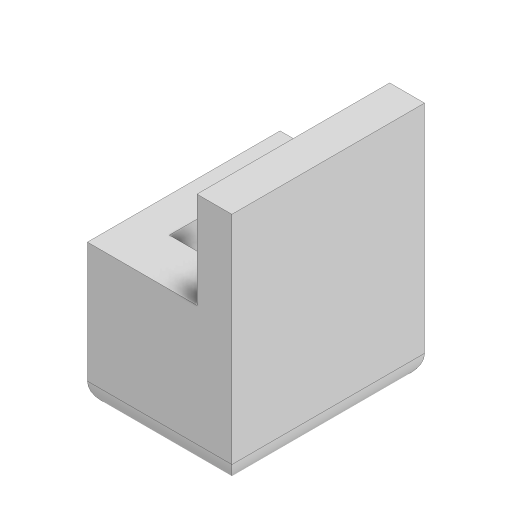
# Autodesk Inventor part: SEGURO DE GUIA DE TAPA PRINCIPAL
Saved by Autodesk Inventor 2024 (Build 280153000, 153)
## iProperties
Created: 2024-09-04
Part Number: SEGURO DE GUIA DE TAPA PRINCIPAL
Material: Generic
Document SubType Name: Modeling
Designer: Jhuliams
Density: 1 g/cm^3
Appearance: Default
Author: Jhuliams
Autodesk Inventor part; units mm, degrees
ref_plane "YZ Plane" through (0, 0, 0) normal (1, 0, 0) x (0, 1, 0)
ref_plane "XZ Plane" through (0, 0, 0) normal (0, 1, 0) x (-1, 0, 0)
ref_plane "XY Plane" through (0, 0, 0) normal (0, 0, 1) x (1, 0, 0)
sketch "Sketch1" plane through (0, 0, 0) normal (0, 1, 0) x (-1, 0, 0)
  line L0 (15, 20) -> (-15, 20)
  line L1 (-15, 20) -> (-15, -20)
  line L2 (-15, -20) -> (15, -20)
  line L3 (15, -20) -> (15, 20)
  line L4 (15, 20) -> (-15, -20) construction
  line L5 (-15, 20) -> (15, -20) construction
  point P0 (0, 0)
  dimension "d0" = 30
  dimension "d1" = 40
  constraints: 12 end point, 2 midpoint, 2 parallel, 1 horizontal, 1 perpendicular
  measures "d0" distance of L2.end L1.end
  measures "d1" distance of L1.end L0.end
extrude "Extrusion1" add sketch "Sketch1" along normal blind 50
sketch "Sketch2" plane through (0, 50, 0) normal (0, 1, 0) x (1, 0, 0)
  line L0 (-7.75, -25.4) -> (7.75, -25.4)
  line L1 (7.75, -25.4) -> (7.75, 25.4)
  line L2 (7.75, 25.4) -> (-7.75, 25.4)
  line L3 (-7.75, 25.4) -> (-7.75, -25.4)
  line L4 (-7.75, -25.4) -> (7.75, 25.4) construction
  line L5 (7.75, -25.4) -> (-7.75, 25.4) construction
  point P0 (0, 0)
  dimension "d4" = 15.5
  constraints: 12 end point, 2 midpoint, 2 parallel, 1 horizontal, 1 perpendicular
  measures "d4" distance of L2.end L1.end
extrude "Extrusion2" cut sketch "Sketch2" against normal blind 20
sketch "Sketch3" plane through (0, 30, 0) normal (0, 1, 0) x (1, 0, 0)
  line L0 (-7.75, -10.25) -> (7.75, -10.25)
  line L1 (7.75, -10.25) -> (7.75, 10.25)
  line L2 (7.75, 10.25) -> (-7.75, 10.25)
  line L3 (-7.75, 10.25) -> (-7.75, -10.25)
  line L4 (-7.75, -10.25) -> (7.75, 10.25) construction
  line L5 (7.75, -10.25) -> (-7.75, 10.25) construction
  point P0 (0, 0)
  dimension "d7" = 15.5
  dimension "d8" = 20.5
  constraints: 12 end point, 2 midpoint, 2 parallel, 1 horizontal, 1 perpendicular
  measures "d7" distance of L2.end L1.end
  measures "d8" distance of L1.end L0.end
extrude "Extrusion3" cut sketch "Sketch3" against normal blind 20.3
fillet "Fillet1" radius 5 4 edges at (15, 0, 0) (-15, 0, 0) (0, 0, 20) (0, 0, -20)
sketch "Sketch4" plane through (0, 50, 0) normal (0, 1, 0) x (1, 0, 0)
  line L0 (-7.75, -20) -> (-7.75, 20) projected
  line L1 (-7.75, 20) -> (-15, 20) projected
  line L2 (-15, 20) -> (-15, -20) projected
  line L3 (-15, -20) -> (-7.75, -20) projected
  point P0 (0, 0)
extrude "Extrusion4" cut sketch "Sketch4" against normal blind 20
body "Solid1"
